Autodesk Fusion 360 part; units mm, degrees
(part 17 of 18)
  line L10453 (179.7854, -37.8851) -> (177.0854, -37.8851)
  line L10454 (177.0854, -39.5851) -> (179.7854, -39.5851)
  line L10455 (177.0854, -37.8851) -> (177.0854, -39.5851)
  line L10456 (103.5852, -77.7106) -> (103.5852, -76.0106)
  line L10457 (100.8852, -76.0106) -> (100.8852, -77.7106)
  line L10458 (100.8852, -77.7106) -> (103.5852, -77.7106)
  line L10459 (103.5852, -76.0106) -> (100.8852, -76.0106)
  line L10460 (103.5852, -56.9478) -> (100.8852, -56.9478)
  line L10461 (103.5852, -58.6478) -> (103.5852, -56.9478)
  line L10462 (100.8852, -56.9478) -> (100.8852, -58.6478)
  line L10463 (100.8852, -58.6478) -> (103.5852, -58.6478)
  line L10464 (103.5852, -20.535) -> (103.5852, -18.835)
  line L10465 (103.5852, -18.835) -> (100.8852, -18.835)
  line L10466 (100.8852, -18.835) -> (100.8852, -20.535)
  line L10467 (100.8852, -20.535) -> (103.5852, -20.535)
  line L10468 (103.5852, -39.5851) -> (103.5852, -37.8851)
  line L10469 (100.8852, -39.5851) -> (103.5852, -39.5851)
  line L10470 (100.8852, -37.8851) -> (100.8852, -39.5851)
  line L10471 (103.5852, -37.8851) -> (100.8852, -37.8851)
  line L10472 (122.6352, -20.535) -> (122.6352, -18.835)
  line L10473 (119.9352, -20.535) -> (122.6352, -20.535)
  line L10474 (122.6352, -18.835) -> (119.9352, -18.835)
  line L10475 (119.9352, -18.835) -> (119.9352, -20.535)
  line L10476 (122.6352, -58.6478) -> (122.6352, -56.9478)
  line L10477 (122.6352, -56.9478) -> (119.9352, -56.9478)
  line L10478 (119.9352, -56.9478) -> (119.9352, -58.6478)
  line L10479 (119.9352, -58.6478) -> (122.6352, -58.6478)
  line L10480 (119.9352, -39.5851) -> (122.6352, -39.5851)
  line L10481 (122.6352, -37.8851) -> (119.9352, -37.8851)
  line L10482 (119.9352, -37.8851) -> (119.9352, -39.5851)
  line L10483 (122.6352, -39.5851) -> (122.6352, -37.8851)
  line L10484 (122.6352, -76.0106) -> (119.9352, -76.0106)
  line L10485 (119.9352, -77.7106) -> (122.6352, -77.7106)
  line L10486 (119.9352, -76.0106) -> (119.9352, -77.7106)
  line L10487 (122.6352, -77.7106) -> (122.6352, -76.0106)
  line L10488 (5.635, -76.0106) -> (5.635, -77.7106)
  line L10489 (8.335, -76.0106) -> (5.635, -76.0106)
  line L10490 (5.635, -77.7106) -> (8.335, -77.7106)
  line L10491 (8.335, -77.7106) -> (8.335, -76.0106)
  line L10492 (24.6851, -77.7106) -> (27.3851, -77.7106)
  line L10493 (24.6851, -76.0106) -> (24.6851, -77.7106)
  line L10494 (27.3851, -76.0106) -> (24.6851, -76.0106)
  line L10495 (27.3851, -77.7106) -> (27.3851, -76.0106)
  line L10496 (43.7351, -77.7106) -> (46.4351, -77.7106)
  line L10497 (46.4351, -77.7106) -> (46.4351, -76.0106)
  line L10498 (43.7351, -76.0106) -> (43.7351, -77.7106)
  line L10499 (46.4351, -76.0106) -> (43.7351, -76.0106)
  line L10500 (62.7851, -18.835) -> (62.7851, -20.535)
  line L10501 (65.4851, -20.535) -> (65.4851, -18.835)
  line L10502 (62.7851, -20.535) -> (65.4851, -20.535)
  line L10503 (65.4851, -18.835) -> (62.7851, -18.835)
  line L10504 (62.7851, -77.7106) -> (65.4851, -77.7106)
  line L10505 (62.7851, -76.0106) -> (62.7851, -77.7106)
  line L10506 (65.4851, -77.7106) -> (65.4851, -76.0106)
  line L10507 (65.4851, -76.0106) -> (62.7851, -76.0106)
  line L10508 (65.4851, -39.5851) -> (65.4851, -37.8851)
  line L10509 (62.7851, -39.5851) -> (65.4851, -39.5851)
  line L10510 (65.4851, -37.8851) -> (62.7851, -37.8851)
  line L10511 (62.7851, -37.8851) -> (62.7851, -39.5851)
  line L10512 (62.7851, -56.9478) -> (62.7851, -58.6478)
  line L10513 (65.4851, -56.9478) -> (62.7851, -56.9478)
  line L10514 (65.4851, -58.6478) -> (65.4851, -56.9478)
  line L10515 (62.7851, -58.6478) -> (65.4851, -58.6478)
  line L10516 (84.5352, -39.5851) -> (84.5352, -37.8851)
  line L10517 (84.5352, -37.8851) -> (81.8352, -37.8851)
  line L10518 (81.8352, -37.8851) -> (81.8352, -39.5851)
  line L10519 (81.8352, -39.5851) -> (84.5352, -39.5851)
  line L10520 (81.8352, -76.0106) -> (81.8352, -77.7106)
  line L10521 (84.5352, -77.7106) -> (84.5352, -76.0106)
  line L10522 (81.8352, -77.7106) -> (84.5352, -77.7106)
  line L10523 (84.5352, -76.0106) -> (81.8352, -76.0106)
  line L10524 (81.8352, -18.835) -> (81.8352, -20.535)
  line L10525 (84.5352, -20.535) -> (84.5352, -18.835)
  line L10526 (84.5352, -18.835) -> (81.8352, -18.835)
  line L10527 (81.8352, -20.535) -> (84.5352, -20.535)
  line L10528 (81.8352, -56.9478) -> (81.8352, -58.6478)
  line L10529 (84.5352, -58.6478) -> (84.5352, -56.9478)
  line L10530 (84.5352, -56.9478) -> (81.8352, -56.9478)
  line L10531 (81.8352, -58.6478) -> (84.5352, -58.6478)
  line L10532 (8.335, -56.9478) -> (5.635, -56.9478)
  line L10533 (5.635, -56.9478) -> (5.635, -58.6478)
  line L10534 (8.335, -58.6478) -> (8.335, -56.9478)
  line L10535 (5.635, -58.6478) -> (8.335, -58.6478)
  line L10536 (8.335, -18.835) -> (5.635, -18.835)
  line L10537 (5.635, -20.535) -> (8.335, -20.535)
  line L10538 (8.335, -20.535) -> (8.335, -18.835)
  line L10539 (5.635, -18.835) -> (5.635, -20.535)
  line L10540 (8.335, -37.8851) -> (5.635, -37.8851)
  line L10541 (8.335, -39.5851) -> (8.335, -37.8851)
  line L10542 (5.635, -37.8851) -> (5.635, -39.5851)
  line L10543 (5.635, -39.5851) -> (8.335, -39.5851)
  line L10544 (27.3851, -37.8851) -> (24.6851, -37.8851)
  line L10545 (24.6851, -37.8851) -> (24.6851, -39.5851)
  line L10546 (27.3851, -39.5851) -> (27.3851, -37.8851)
  line L10547 (24.6851, -39.5851) -> (27.3851, -39.5851)
  line L10548 (27.3851, -18.835) -> (24.6851, -18.835)
  line L10549 (27.3851, -20.535) -> (27.3851, -18.835)
  line L10550 (24.6851, -20.535) -> (27.3851, -20.535)
  line L10551 (24.6851, -18.835) -> (24.6851, -20.535)
  line L10552 (24.6851, -56.9478) -> (24.6851, -58.6478)
  line L10553 (24.6851, -58.6478) -> (27.3851, -58.6478)
  line L10554 (27.3851, -56.9478) -> (24.6851, -56.9478)
  line L10555 (27.3851, -58.6478) -> (27.3851, -56.9478)
  line L10556 (46.4351, -18.835) -> (43.7351, -18.835)
  line L10557 (43.7351, -18.835) -> (43.7351, -20.535)
  line L10558 (46.4351, -20.535) -> (46.4351, -18.835)
  line L10559 (43.7351, -20.535) -> (46.4351, -20.535)
  line L10560 (43.7351, -58.6478) -> (46.4351, -58.6478)
  line L10561 (46.4351, -58.6478) -> (46.4351, -56.9478)
  line L10562 (46.4351, -56.9478) -> (43.7351, -56.9478)
  line L10563 (43.7351, -56.9478) -> (43.7351, -58.6478)
  line L10564 (43.7351, -39.5851) -> (46.4351, -39.5851)
  line L10565 (43.7351, -37.8851) -> (43.7351, -39.5851)
  line L10566 (46.4351, -39.5851) -> (46.4351, -37.8851)
  line L10567 (46.4351, -37.8851) -> (43.7351, -37.8851)
  line L10568 (215.1854, -18.835) -> (215.1854, -20.535)
  line L10569 (217.8854, -18.835) -> (215.1854, -18.835)
  line L10570 (217.8854, -20.535) -> (217.8854, -18.835)
  line L10571 (215.1854, -20.535) -> (217.8854, -20.535)
  line L10572 (217.8854, -76.0106) -> (215.1854, -76.0106)
  line L10573 (217.8854, -77.7106) -> (217.8854, -76.0106)
  line L10574 (215.1854, -77.7106) -> (217.8854, -77.7106)
  line L10575 (215.1854, -76.0106) -> (215.1854, -77.7106)
  line L10576 (215.1854, -58.6478) -> (217.8854, -58.6478)
  line L10577 (217.8854, -56.9478) -> (215.1854, -56.9478)
  line L10578 (217.8854, -58.6478) -> (217.8854, -56.9478)
  line L10579 (215.1854, -56.9478) -> (215.1854, -58.6478)
  line L10580 (215.1854, -37.8851) -> (215.1854, -39.5851)
  line L10581 (217.8854, -39.5851) -> (217.8854, -37.8851)
  line L10582 (215.1854, -39.5851) -> (217.8854, -39.5851)
  line L10583 (217.8854, -37.8851) -> (215.1854, -37.8851)
  line L10584 (196.1354, -37.8851) -> (196.1354, -39.5851)
  line L10585 (196.1354, -39.5851) -> (198.8354, -39.5851)
  line L10586 (198.8354, -39.5851) -> (198.8354, -37.8851)
  line L10587 (198.8354, -37.8851) -> (196.1354, -37.8851)
  line L10588 (198.8354, -76.0106) -> (196.1354, -76.0106)
  line L10589 (198.8354, -77.7106) -> (198.8354, -76.0106)
  line L10590 (196.1354, -76.0106) -> (196.1354, -77.7106)
  line L10591 (196.1354, -77.7106) -> (198.8354, -77.7106)
  line L10592 (196.1354, -56.9478) -> (196.1354, -58.6478)
  line L10593 (196.1354, -58.6478) -> (198.8354, -58.6478)
  line L10594 (198.8354, -56.9478) -> (196.1354, -56.9478)
  line L10595 (198.8354, -58.6478) -> (198.8354, -56.9478)
  line L10596 (196.1354, -18.835) -> (196.1354, -20.535)
  line L10597 (196.1354, -20.535) -> (198.8354, -20.535)
  line L10598 (198.8354, -18.835) -> (196.1354, -18.835)
  line L10599 (198.8354, -20.535) -> (198.8354, -18.835)
  line L10600 (203.2384, -4.21) -> (201.6384, -4.21)
  line L10601 (201.6384, -4.21) -> (201.6384, -3.41)
  line L10602 (201.6384, -3.41) -> (203.2384, -3.41)
  line L10603 (203.2384, -3.41) -> (203.2384, -4.21)
  line L10604 (199.7334, -7.131) -> (199.7334, -6.331)
  line L10605 (199.7334, -6.331) -> (201.3334, -6.331)
  line L10606 (201.3334, -7.131) -> (199.7334, -7.131)
  line L10607 (201.3334, -6.331) -> (201.3334, -7.131)
  line L10608 (206.5404, -4.426) -> (206.5404, -5.226)
  line L10609 (204.9404, -4.426) -> (206.5404, -4.426)
  line L10610 (206.5404, -5.226) -> (204.9404, -5.226)
  line L10611 (204.9404, -5.226) -> (204.9404, -4.426)
  line L10612 (-5.7371, 1.189) -> (10.5631, 1.189)
  line L10613 (10.5631, -12.111) -> (-5.7371, -12.111)
  line L10614 (-5.7371, -12.111) -> (-5.7371, 1.189)
  line L10615 (10.5631, 1.189) -> (10.5631, -12.111)
  line L10616 (196.9574, -3.429) -> (196.9574, -5.529)
  line L10617 (195.7074, -5.529) -> (195.7074, -3.429)
  line L10618 (195.7074, -3.429) -> (196.9574, -3.429)
  line L10619 (196.9574, -5.529) -> (195.7074, -5.529)
  line L10620 (177.1673, -5.588) -> (172.3373, -5.588)
  line L10621 (172.3373, -3.048) -> (177.1673, -3.048)
  line L10622 (172.3373, -5.588) -> (172.3373, -3.048)
  line L10623 (177.1673, -3.048) -> (177.1673, -5.588)
  line L10624 (199.8604, -1.505) -> (201.4604, -1.505)
  line L10625 (201.4604, -1.505) -> (201.4604, -2.305)
  line L10626 (201.4604, -2.305) -> (199.8604, -2.305)
  line L10627 (199.8604, -2.305) -> (199.8604, -1.505)
  line L10628 (214.5745, -5.2629) -> (214.5745, -12.2629)
  line L10629 (214.5745, -12.2629) -> (207.5745, -12.2629)
  line L10630 (207.5745, -5.2629) -> (214.5745, -5.2629)
  line L10631 (207.5745, -12.2629) -> (207.5745, -5.2629)
  line L10632 (188.5064, -6.331) -> (188.5064, -7.131)
  line L10633 (186.9064, -6.331) -> (188.5064, -6.331)
  line L10634 (188.5064, -7.131) -> (186.9064, -7.131)
  line L10635 (186.9064, -7.131) -> (186.9064, -6.331)
  line L10636 (182.3344, -7.131) -> (182.3344, -6.331)
  line L10637 (183.9344, -7.131) -> (182.3344, -7.131)
  line L10638 (183.9344, -6.331) -> (183.9344, -7.131)
  line L10639 (182.3344, -6.331) -> (183.9344, -6.331)
  line L10640 (208.6854, -0.786) -> (211.6854, -0.786)
  line L10641 (208.6854, -3.786) -> (208.6854, -0.786)
  line L10642 (211.6854, -3.786) -> (208.6854, -3.786)
  line L10643 (211.6854, -0.786) -> (211.6854, -3.786)
  line L10644 (138.9853, -77.7106) -> (141.6853, -77.7106)
  line L10645 (138.9853, -76.0106) -> (138.9853, -77.7106)
  line L10646 (141.6853, -76.0106) -> (138.9853, -76.0106)
  line L10647 (141.6853, -77.7106) -> (141.6853, -76.0106)
  line L10648 (138.9853, -20.535) -> (141.6853, -20.535)
  line L10649 (141.6853, -20.535) -> (141.6853, -18.835)
  line L10650 (141.6853, -18.835) -> (138.9853, -18.835)
  line L10651 (138.9853, -18.835) -> (138.9853, -20.535)
  line L10652 (138.9853, -39.5851) -> (141.6853, -39.5851)
  line L10653 (141.6853, -37.8851) -> (138.9853, -37.8851)
  line L10654 (138.9853, -37.8851) -> (138.9853, -39.5851)
  line L10655 (141.6853, -39.5851) -> (141.6853, -37.8851)
  line L10656 (138.9853, -56.9478) -> (138.9853, -58.6478)
  line L10657 (141.6853, -56.9478) -> (138.9853, -56.9478)
  line L10658 (138.9853, -58.6478) -> (141.6853, -58.6478)
  line L10659 (141.6853, -58.6478) -> (141.6853, -56.9478)
  line L10660 (158.0353, -20.535) -> (160.7353, -20.535)
  line L10661 (160.7353, -18.835) -> (158.0353, -18.835)
  line L10662 (160.7353, -20.535) -> (160.7353, -18.835)
  line L10663 (158.0353, -18.835) -> (158.0353, -20.535)
  line L10664 (158.0353, -76.0106) -> (158.0353, -77.7106)
  line L10665 (160.7353, -76.0106) -> (158.0353, -76.0106)
  line L10666 (158.0353, -77.7106) -> (160.7353, -77.7106)
  line L10667 (160.7353, -77.7106) -> (160.7353, -76.0106)
  line L10668 (158.0353, -56.9478) -> (158.0353, -58.6478)
  line L10669 (160.7353, -58.6478) -> (160.7353, -56.9478)
  line L10670 (160.7353, -56.9478) -> (158.0353, -56.9478)
  line L10671 (158.0353, -58.6478) -> (160.7353, -58.6478)
  line L10672 (160.7353, -39.5851) -> (160.7353, -37.8851)
  line L10673 (160.7353, -37.8851) -> (158.0353, -37.8851)
  line L10674 (158.0353, -39.5851) -> (160.7353, -39.5851)
  line L10675 (158.0353, -37.8851) -> (158.0353, -39.5851)
  line L10676 (177.0854, -20.535) -> (179.7854, -20.535)
  line L10677 (179.7854, -18.835) -> (177.0854, -18.835)
  line L10678 (179.7854, -20.535) -> (179.7854, -18.835)
  line L10679 (177.0854, -18.835) -> (177.0854, -20.535)
  line L10680 (177.0854, -76.0106) -> (177.0854, -77.7106)
  line L10681 (179.7854, -77.7106) -> (179.7854, -76.0106)
  line L10682 (177.0854, -77.7106) -> (179.7854, -77.7106)
  line L10683 (179.7854, -76.0106) -> (177.0854, -76.0106)
  line L10684 (177.0854, -56.9478) -> (177.0854, -58.6478)
  line L10685 (177.0854, -58.6478) -> (179.7854, -58.6478)
  line L10686 (179.7854, -58.6478) -> (179.7854, -56.9478)
  line L10687 (179.7854, -56.9478) -> (177.0854, -56.9478)
  line L10688 (177.0854, -37.8851) -> (177.0854, -39.5851)
  line L10689 (177.0854, -39.5851) -> (179.7854, -39.5851)
  line L10690 (179.7854, -39.5851) -> (179.7854, -37.8851)
  line L10691 (179.7854, -37.8851) -> (177.0854, -37.8851)
  line L10692 (103.5852, -77.7106) -> (103.5852, -76.0106)
  line L10693 (100.8852, -76.0106) -> (100.8852, -77.7106)
  line L10694 (103.5852, -76.0106) -> (100.8852, -76.0106)
  line L10695 (100.8852, -77.7106) -> (103.5852, -77.7106)
  line L10696 (103.5852, -58.6478) -> (103.5852, -56.9478)
  line L10697 (103.5852, -56.9478) -> (100.8852, -56.9478)
  line L10698 (100.8852, -56.9478) -> (100.8852, -58.6478)
  line L10699 (100.8852, -58.6478) -> (103.5852, -58.6478)
  line L10700 (100.8852, -20.535) -> (103.5852, -20.535)
  line L10701 (100.8852, -18.835) -> (100.8852, -20.535)
  line L10702 (103.5852, -20.535) -> (103.5852, -18.835)
  line L10703 (103.5852, -18.835) -> (100.8852, -18.835)
  line L10704 (103.5852, -39.5851) -> (103.5852, -37.8851)
  line L10705 (100.8852, -37.8851) -> (100.8852, -39.5851)
  line L10706 (100.8852, -39.5851) -> (103.5852, -39.5851)
  line L10707 (103.5852, -37.8851) -> (100.8852, -37.8851)
  line L10708 (122.6352, -18.835) -> (119.9352, -18.835)
  line L10709 (119.9352, -18.835) -> (119.9352, -20.535)
  line L10710 (119.9352, -20.535) -> (122.6352, -20.535)
  line L10711 (122.6352, -20.535) -> (122.6352, -18.835)
  line L10712 (119.9352, -58.6478) -> (122.6352, -58.6478)
  line L10713 (122.6352, -56.9478) -> (119.9352, -56.9478)
  line L10714 (122.6352, -58.6478) -> (122.6352, -56.9478)
  line L10715 (119.9352, -56.9478) -> (119.9352, -58.6478)
  line L10716 (122.6352, -39.5851) -> (122.6352, -37.8851)
  line L10717 (119.9352, -39.5851) -> (122.6352, -39.5851)
  line L10718 (119.9352, -37.8851) -> (119.9352, -39.5851)
  line L10719 (122.6352, -37.8851) -> (119.9352, -37.8851)
  line L10720 (122.6352, -76.0106) -> (119.9352, -76.0106)
  line L10721 (122.6352, -77.7106) -> (122.6352, -76.0106)
  line L10722 (119.9352, -76.0106) -> (119.9352, -77.7106)
  line L10723 (119.9352, -77.7106) -> (122.6352, -77.7106)
  line L10724 (5.635, -76.0106) -> (5.635, -77.7106)
  line L10725 (8.335, -77.7106) -> (8.335, -76.0106)
  line L10726 (5.635, -77.7106) -> (8.335, -77.7106)
  line L10727 (8.335, -76.0106) -> (5.635, -76.0106)
  line L10728 (27.3851, -76.0106) -> (24.6851, -76.0106)
  line L10729 (27.3851, -77.7106) -> (27.3851, -76.0106)
  line L10730 (24.6851, -76.0106) -> (24.6851, -77.7106)
  line L10731 (24.6851, -77.7106) -> (27.3851, -77.7106)
  line L10732 (46.4351, -76.0106) -> (43.7351, -76.0106)
  line L10733 (43.7351, -77.7106) -> (46.4351, -77.7106)
  line L10734 (46.4351, -77.7106) -> (46.4351, -76.0106)
  line L10735 (43.7351, -76.0106) -> (43.7351, -77.7106)
  line L10736 (62.7851, -20.535) -> (65.4851, -20.535)
  line L10737 (65.4851, -20.535) -> (65.4851, -18.835)
  line L10738 (62.7851, -18.835) -> (62.7851, -20.535)
  line L10739 (65.4851, -18.835) -> (62.7851, -18.835)
  line L10740 (62.7851, -76.0106) -> (62.7851, -77.7106)
  line L10741 (65.4851, -76.0106) -> (62.7851, -76.0106)
  line L10742 (62.7851, -77.7106) -> (65.4851, -77.7106)
  line L10743 (65.4851, -77.7106) -> (65.4851, -76.0106)
  line L10744 (62.7851, -39.5851) -> (65.4851, -39.5851)
  line L10745 (65.4851, -39.5851) -> (65.4851, -37.8851)
  line L10746 (65.4851, -37.8851) -> (62.7851, -37.8851)
  line L10747 (62.7851, -37.8851) -> (62.7851, -39.5851)
  line L10748 (62.7851, -58.6478) -> (65.4851, -58.6478)
  line L10749 (62.7851, -56.9478) -> (62.7851, -58.6478)
  line L10750 (65.4851, -58.6478) -> (65.4851, -56.9478)
  line L10751 (65.4851, -56.9478) -> (62.7851, -56.9478)
  line L10752 (84.5352, -39.5851) -> (84.5352, -37.8851)
  line L10753 (81.8352, -37.8851) -> (81.8352, -39.5851)
  line L10754 (81.8352, -39.5851) -> (84.5352, -39.5851)
  line L10755 (84.5352, -37.8851) -> (81.8352, -37.8851)
  line L10756 (84.5352, -77.7106) -> (84.5352, -76.0106)
  line L10757 (81.8352, -76.0106) -> (81.8352, -77.7106)
  line L10758 (81.8352, -77.7106) -> (84.5352, -77.7106)
  line L10759 (84.5352, -76.0106) -> (81.8352, -76.0106)
  line L10760 (84.5352, -20.535) -> (84.5352, -18.835)
  line L10761 (84.5352, -18.835) -> (81.8352, -18.835)
  line L10762 (81.8352, -20.535) -> (84.5352, -20.535)
  line L10763 (81.8352, -18.835) -> (81.8352, -20.535)
  line L10764 (81.8352, -58.6478) -> (84.5352, -58.6478)
  line L10765 (81.8352, -56.9478) -> (81.8352, -58.6478)
  line L10766 (84.5352, -56.9478) -> (81.8352, -56.9478)
  line L10767 (84.5352, -58.6478) -> (84.5352, -56.9478)
  line L10768 (5.635, -58.6478) -> (8.335, -58.6478)
  line L10769 (8.335, -56.9478) -> (5.635, -56.9478)
  line L10770 (5.635, -56.9478) -> (5.635, -58.6478)
  line L10771 (8.335, -58.6478) -> (8.335, -56.9478)
  line L10772 (8.335, -20.535) -> (8.335, -18.835)
  line L10773 (8.335, -18.835) -> (5.635, -18.835)
  line L10774 (5.635, -18.835) -> (5.635, -20.535)
  line L10775 (5.635, -20.535) -> (8.335, -20.535)
  line L10776 (8.335, -37.8851) -> (5.635, -37.8851)
  line L10777 (5.635, -39.5851) -> (8.335, -39.5851)
  line L10778 (5.635, -37.8851) -> (5.635, -39.5851)
  line L10779 (8.335, -39.5851) -> (8.335, -37.8851)
  line L10780 (27.3851, -37.8851) -> (24.6851, -37.8851)
  line L10781 (24.6851, -39.5851) -> (27.3851, -39.5851)
  line L10782 (24.6851, -37.8851) -> (24.6851, -39.5851)
  line L10783 (27.3851, -39.5851) -> (27.3851, -37.8851)
  line L10784 (24.6851, -20.535) -> (27.3851, -20.535)
  line L10785 (27.3851, -20.535) -> (27.3851, -18.835)
  line L10786 (24.6851, -18.835) -> (24.6851, -20.535)
  line L10787 (27.3851, -18.835) -> (24.6851, -18.835)
  line L10788 (24.6851, -56.9478) -> (24.6851, -58.6478)
  line L10789 (27.3851, -56.9478) -> (24.6851, -56.9478)
  line L10790 (24.6851, -58.6478) -> (27.3851, -58.6478)
  line L10791 (27.3851, -58.6478) -> (27.3851, -56.9478)
  line L10792 (43.7351, -20.535) -> (46.4351, -20.535)
  line L10793 (43.7351, -18.835) -> (43.7351, -20.535)
  line L10794 (46.4351, -20.535) -> (46.4351, -18.835)
  line L10795 (46.4351, -18.835) -> (43.7351, -18.835)
  line L10796 (43.7351, -58.6478) -> (46.4351, -58.6478)
  line L10797 (46.4351, -58.6478) -> (46.4351, -56.9478)
  line L10798 (46.4351, -56.9478) -> (43.7351, -56.9478)
  line L10799 (43.7351, -56.9478) -> (43.7351, -58.6478)
  line L10800 (46.4351, -37.8851) -> (43.7351, -37.8851)
  line L10801 (43.7351, -39.5851) -> (46.4351, -39.5851)
  line L10802 (43.7351, -37.8851) -> (43.7351, -39.5851)
  line L10803 (46.4351, -39.5851) -> (46.4351, -37.8851)
  line L10804 (217.8854, -20.535) -> (217.8854, -18.835)
  line L10805 (217.8854, -18.835) -> (215.1854, -18.835)
  line L10806 (215.1854, -18.835) -> (215.1854, -20.535)
  line L10807 (215.1854, -20.535) -> (217.8854, -20.535)
  line L10808 (215.1854, -77.7106) -> (217.8854, -77.7106)
  line L10809 (215.1854, -76.0106) -> (215.1854, -77.7106)
  line L10810 (217.8854, -76.0106) -> (215.1854, -76.0106)
  line L10811 (217.8854, -77.7106) -> (217.8854, -76.0106)
  line L10812 (217.8854, -56.9478) -> (215.1854, -56.9478)
  line L10813 (215.1854, -58.6478) -> (217.8854, -58.6478)
  line L10814 (217.8854, -58.6478) -> (217.8854, -56.9478)
  line L10815 (215.1854, -56.9478) -> (215.1854, -58.6478)
  line L10816 (217.8854, -37.8851) -> (215.1854, -37.8851)
  line L10817 (215.1854, -37.8851) -> (215.1854, -39.5851)
  line L10818 (217.8854, -39.5851) -> (217.8854, -37.8851)
  line L10819 (215.1854, -39.5851) -> (217.8854, -39.5851)
  line L10820 (198.8354, -37.8851) -> (196.1354, -37.8851)
  line L10821 (196.1354, -37.8851) -> (196.1354, -39.5851)
  line L10822 (196.1354, -39.5851) -> (198.8354, -39.5851)
  line L10823 (198.8354, -39.5851) -> (198.8354, -37.8851)
  line L10824 (196.1354, -77.7106) -> (198.8354, -77.7106)
  line L10825 (196.1354, -76.0106) -> (196.1354, -77.7106)
  line L10826 (198.8354, -76.0106) -> (196.1354, -76.0106)
  line L10827 (198.8354, -77.7106) -> (198.8354, -76.0106)
  line L10828 (196.1354, -58.6478) -> (198.8354, -58.6478)
  line L10829 (196.1354, -56.9478) -> (196.1354, -58.6478)
  line L10830 (198.8354, -58.6478) -> (198.8354, -56.9478)
  line L10831 (198.8354, -56.9478) -> (196.1354, -56.9478)
  line L10832 (198.8354, -20.535) -> (198.8354, -18.835)
  line L10833 (196.1354, -20.535) -> (198.8354, -20.535)
  line L10834 (198.8354, -18.835) -> (196.1354, -18.835)
  line L10835 (196.1354, -18.835) -> (196.1354, -20.535)
  line L10836 (201.6384, -3.41) -> (203.2384, -3.41)
  line L10837 (201.6384, -4.21) -> (201.6384, -3.41)
  line L10838 (203.2384, -3.41) -> (203.2384, -4.21)
  line L10839 (203.2384, -4.21) -> (201.6384, -4.21)
  line L10840 (199.7334, -6.331) -> (201.3334, -6.331)
  line L10841 (201.3334, -7.131) -> (199.7334, -7.131)
  line L10842 (199.7334, -7.131) -> (199.7334, -6.331)
  line L10843 (201.3334, -6.331) -> (201.3334, -7.131)
  line L10844 (204.9404, -4.426) -> (206.5404, -4.426)
  line L10845 (206.5404, -4.426) -> (206.5404, -5.226)
  line L10846 (204.9404, -5.226) -> (204.9404, -4.426)
  line L10847 (206.5404, -5.226) -> (204.9404, -5.226)
  line L10848 (-5.7371, -12.111) -> (-5.7371, 1.189)
  line L10849 (10.5631, 1.189) -> (10.5631, -12.111)
  line L10850 (10.5631, -12.111) -> (-5.7371, -12.111)
  line L10851 (-5.7371, 1.189) -> (10.5631, 1.189)
  line L10852 (195.7074, -5.529) -> (195.7074, -3.429)
  line L10853 (195.7074, -3.429) -> (196.9574, -3.429)
  line L10854 (196.9574, -5.529) -> (195.7074, -5.529)
  line L10855 (196.9574, -3.429) -> (196.9574, -5.529)
  line L10856 (177.1673, -5.588) -> (172.3373, -5.588)
  line L10857 (177.1673, -3.048) -> (177.1673, -5.588)
  line L10858 (172.3373, -3.048) -> (177.1673, -3.048)
  line L10859 (172.3373, -5.588) -> (172.3373, -3.048)
  line L10860 (208.2754, -3.1661) -> (208.6954, -3.1661)
  line L10861 (208.6954, -3.1661) -> (208.6954, -3.4061)
  line L10862 (208.6954, -3.4061) -> (208.2754, -3.4061)
  line L10863 (208.2754, -3.4061) -> (208.2754, -3.1661)
  line L10864 (208.6954, -2.666) -> (208.6954, -2.906)
  line L10865 (208.2754, -2.666) -> (208.6954, -2.666)
  line L10866 (208.2754, -2.906) -> (208.2754, -2.666)
  line L10867 (208.6954, -2.906) -> (208.2754, -2.906)
  line L10868 (208.2754, -2.1659) -> (208.6954, -2.1659)
  line L10869 (208.2754, -2.4059) -> (208.2754, -2.1659)
  line L10870 (208.6954, -2.1659) -> (208.6954, -2.4059)
  line L10871 (208.6954, -2.4059) -> (208.2754, -2.4059)
  line L10872 (208.2754, -1.906) -> (208.2754, -1.666)
  line L10873 (208.2754, -1.666) -> (208.6954, -1.666)
  line L10874 (208.6954, -1.666) -> (208.6954, -1.906)
  line L10875 (208.6954, -1.906) -> (208.2754, -1.906)
  line L10876 (208.6954, -1.4061) -> (208.2754, -1.4061)
  line L10877 (208.2754, -1.4061) -> (208.2754, -1.1661)
  line L10878 (208.6954, -1.1661) -> (208.6954, -1.4061)
  line L10879 (208.2754, -1.1661) -> (208.6954, -1.1661)
  line L10880 (212.0954, -1.4059) -> (211.6754, -1.4059)
  line L10881 (211.6754, -1.1659) -> (212.0954, -1.1659)
  line L10882 (212.0954, -1.1659) -> (212.0954, -1.4059)
  line L10883 (211.6754, -1.4059) -> (211.6754, -1.1659)
  line L10884 (211.6754, -1.906) -> (211.6754, -1.666)
  line L10885 (212.0954, -1.906) -> (211.6754, -1.906)
  line L10886 (212.0954, -1.666) -> (212.0954, -1.906)
  line L10887 (211.6754, -1.666) -> (212.0954, -1.666)
  line L10888 (212.0954, -2.4061) -> (211.6754, -2.4061)
  line L10889 (212.0954, -2.1661) -> (212.0954, -2.4061)
  line L10890 (211.6754, -2.4061) -> (211.6754, -2.1661)
  line L10891 (211.6754, -2.1661) -> (212.0954, -2.1661)
  line L10892 (211.6754, -2.666) -> (212.0954, -2.666)
  line L10893 (212.0954, -2.666) -> (212.0954, -2.906)
  line L10894 (211.6754, -2.906) -> (211.6754, -2.666)
  line L10895 (212.0954, -2.906) -> (211.6754, -2.906)
  line L10896 (211.6754, -3.4059) -> (211.6754, -3.1659)
  line L10897 (211.6754, -3.1659) -> (212.0954, -3.1659)
  line L10898 (212.0954, -3.1659) -> (212.0954, -3.4059)
  line L10899 (212.0954, -3.4059) -> (211.6754, -3.4059)
  line L10900 (138.7753, -77.1606) -> (138.9953, -77.1606)
  line L10901 (138.7753, -76.5606) -> (138.7753, -77.1606)
  line L10902 (138.9953, -76.5606) -> (138.7753, -76.5606)
  line L10903 (138.9953, -77.1606) -> (138.9953, -76.5606)
  line L10904 (141.6753, -76.5606) -> (141.8953, -76.5606)
  line L10905 (141.6753, -77.1606) -> (141.6753, -76.5606)
  line L10906 (141.8953, -77.1606) -> (141.6753, -77.1606)
  line L10907 (141.8953, -76.5606) -> (141.8953, -77.1606)
  line L10908 (138.7753, -19.385) -> (138.7753, -19.985)
  line L10909 (138.9953, -19.385) -> (138.7753, -19.385)
  line L10910 (138.9953, -19.985) -> (138.9953, -19.385)
  line L10911 (138.7753, -19.985) -> (138.9953, -19.985)
  line L10912 (141.8953, -19.985) -> (141.6753, -19.985)
  line L10913 (141.6753, -19.385) -> (141.8953, -19.385)
  line L10914 (141.6753, -19.985) -> (141.6753, -19.385)
  line L10915 (141.8953, -19.385) -> (141.8953, -19.985)
  line L10916 (138.7753, -39.0351) -> (138.9953, -39.0351)
  line L10917 (138.9953, -39.0351) -> (138.9953, -38.4351)
  line L10918 (138.7753, -38.4351) -> (138.7753, -39.0351)
  line L10919 (138.9953, -38.4351) -> (138.7753, -38.4351)
  line L10920 (141.6753, -38.4351) -> (141.8953, -38.4351)
  line L10921 (141.6753, -39.0351) -> (141.6753, -38.4351)
  line L10922 (141.8953, -38.4351) -> (141.8953, -39.0351)
  line L10923 (141.8953, -39.0351) -> (141.6753, -39.0351)
  line L10924 (138.9953, -57.4978) -> (138.7753, -57.4978)
  line L10925 (138.9953, -58.0978) -> (138.9953, -57.4978)
  line L10926 (138.7753, -58.0978) -> (138.9953, -58.0978)
  line L10927 (138.7753, -57.4978) -> (138.7753, -58.0978)
  line L10928 (141.8953, -58.0978) -> (141.6753, -58.0978)
  line L10929 (141.8953, -57.4978) -> (141.8953, -58.0978)
  line L10930 (141.6753, -57.4978) -> (141.8953, -57.4978)
  line L10931 (141.6753, -58.0978) -> (141.6753, -57.4978)
  line L10932 (158.0453, -19.385) -> (157.8253, -19.385)
  line L10933 (157.8253, -19.385) -> (157.8253, -19.985)
  line L10934 (157.8253, -19.985) -> (158.0453, -19.985)
  line L10935 (158.0453, -19.985) -> (158.0453, -19.385)
  line L10936 (160.9453, -19.985) -> (160.7253, -19.985)
  line L10937 (160.7253, -19.985) -> (160.7253, -19.385)
  line L10938 (160.7253, -19.385) -> (160.9453, -19.385)
  line L10939 (160.9453, -19.385) -> (160.9453, -19.985)
  line L10940 (158.0453, -76.5606) -> (157.8253, -76.5606)
  line L10941 (158.0453, -77.1606) -> (158.0453, -76.5606)
  line L10942 (157.8253, -76.5606) -> (157.8253, -77.1606)
  line L10943 (157.8253, -77.1606) -> (158.0453, -77.1606)
  line L10944 (160.7253, -77.1606) -> (160.7253, -76.5606)
  line L10945 (160.9453, -77.1606) -> (160.7253, -77.1606)
  line L10946 (160.7253, -76.5606) -> (160.9453, -76.5606)
  line L10947 (160.9453, -76.5606) -> (160.9453, -77.1606)
  line L10948 (158.0453, -58.0978) -> (158.0453, -57.4978)
  line L10949 (158.0453, -57.4978) -> (157.8253, -57.4978)
  line L10950 (157.8253, -58.0978) -> (158.0453, -58.0978)
  line L10951 (157.8253, -57.4978) -> (157.8253, -58.0978)
  line L10952 (160.7253, -58.0978) -> (160.7253, -57.4978)
  line L10953 (160.7253, -57.4978) -> (160.9453, -57.4978)
  line L10954 (160.9453, -58.0978) -> (160.7253, -58.0978)
  line L10955 (160.9453, -57.4978) -> (160.9453, -58.0978)
  line L10956 (158.0453, -39.0351) -> (158.0453, -38.4351)
  line L10957 (157.8253, -39.0351) -> (158.0453, -39.0351)
  line L10958 (158.0453, -38.4351) -> (157.8253, -38.4351)
  line L10959 (157.8253, -38.4351) -> (157.8253, -39.0351)
  line L10960 (160.7253, -38.4351) -> (160.9453, -38.4351)
  line L10961 (160.9453, -38.4351) -> (160.9453, -39.0351)
  line L10962 (160.9453, -39.0351) -> (160.7253, -39.0351)
  line L10963 (160.7253, -39.0351) -> (160.7253, -38.4351)
  line L10964 (177.0954, -19.985) -> (177.0954, -19.385)
  line L10965 (176.8754, -19.985) -> (177.0954, -19.985)
  line L10966 (176.8754, -19.385) -> (176.8754, -19.985)
  line L10967 (177.0954, -19.385) -> (176.8754, -19.385)
  line L10968 (179.9954, -19.985) -> (179.7754, -19.985)
  line L10969 (179.7754, -19.985) -> (179.7754, -19.385)
  line L10970 (179.7754, -19.385) -> (179.9954, -19.385)
  line L10971 (179.9954, -19.385) -> (179.9954, -19.985)
  line L10972 (176.8754, -76.5606) -> (176.8754, -77.1606)
  line L10973 (177.0954, -76.5606) -> (176.8754, -76.5606)
  line L10974 (176.8754, -77.1606) -> (177.0954, -77.1606)
  line L10975 (177.0954, -77.1606) -> (177.0954, -76.5606)
  line L10976 (179.9954, -77.1606) -> (179.7754, -77.1606)
  line L10977 (179.7754, -76.5606) -> (179.9954, -76.5606)
  line L10978 (179.7754, -77.1606) -> (179.7754, -76.5606)
  line L10979 (179.9954, -76.5606) -> (179.9954, -77.1606)
  line L10980 (177.0954, -57.4978) -> (176.8754, -57.4978)
  line L10981 (176.8754, -58.0978) -> (177.0954, -58.0978)
  line L10982 (176.8754, -57.4978) -> (176.8754, -58.0978)
  line L10983 (177.0954, -58.0978) -> (177.0954, -57.4978)
  line L10984 (179.7754, -57.4978) -> (179.9954, -57.4978)
  line L10985 (179.7754, -58.0978) -> (179.7754, -57.4978)
  line L10986 (179.9954, -57.4978) -> (179.9954, -58.0978)
  line L10987 (179.9954, -58.0978) -> (179.7754, -58.0978)
  line L10988 (177.0954, -39.0351) -> (177.0954, -38.4351)
  line L10989 (176.8754, -39.0351) -> (177.0954, -39.0351)
  line L10990 (176.8754, -38.4351) -> (176.8754, -39.0351)
  line L10991 (177.0954, -38.4351) -> (176.8754, -38.4351)
  line L10992 (179.9954, -38.4351) -> (179.9954, -39.0351)
  line L10993 (179.7754, -38.4351) -> (179.9954, -38.4351)
  line L10994 (179.7754, -39.0351) -> (179.7754, -38.4351)
  line L10995 (179.9954, -39.0351) -> (179.7754, -39.0351)
  line L10996 (100.6752, -76.5606) -> (100.6752, -77.1606)
  line L10997 (100.8952, -77.1606) -> (100.8952, -76.5606)
  line L10998 (100.6752, -77.1606) -> (100.8952, -77.1606)
  line L10999 (100.8952, -76.5606) -> (100.6752, -76.5606)
  line L11000 (103.7952, -77.1606) -> (103.5752, -77.1606)
  line L11001 (103.5752, -77.1606) -> (103.5752, -76.5606)
  line L11002 (103.7952, -76.5606) -> (103.7952, -77.1606)
  line L11003 (103.5752, -76.5606) -> (103.7952, -76.5606)
  line L11004 (100.8952, -57.4978) -> (100.6752, -57.4978)
  line L11005 (100.8952, -58.0978) -> (100.8952, -57.4978)
  line L11006 (100.6752, -58.0978) -> (100.8952, -58.0978)
  line L11007 (100.6752, -57.4978) -> (100.6752, -58.0978)
  line L11008 (103.7952, -57.4978) -> (103.7952, -58.0978)
  line L11009 (103.5752, -58.0978) -> (103.5752, -57.4978)
  line L11010 (103.7952, -58.0978) -> (103.5752, -58.0978)
  line L11011 (103.5752, -57.4978) -> (103.7952, -57.4978)
  line L11012 (100.6752, -19.385) -> (100.6752, -19.985)
  line L11013 (100.8952, -19.985) -> (100.8952, -19.385)
  line L11014 (100.6752, -19.985) -> (100.8952, -19.985)
  line L11015 (100.8952, -19.385) -> (100.6752, -19.385)
  line L11016 (103.5752, -19.385) -> (103.7952, -19.385)
  line L11017 (103.5752, -19.985) -> (103.5752, -19.385)
  line L11018 (103.7952, -19.985) -> (103.5752, -19.985)
  line L11019 (103.7952, -19.385) -> (103.7952, -19.985)
  line L11020 (100.8952, -38.4351) -> (100.6752, -38.4351)
  line L11021 (100.6752, -38.4351) -> (100.6752, -39.0351)
  line L11022 (100.8952, -39.0351) -> (100.8952, -38.4351)
  line L11023 (100.6752, -39.0351) -> (100.8952, -39.0351)
  line L11024 (103.7952, -39.0351) -> (103.5752, -39.0351)
  line L11025 (103.5752, -38.4351) -> (103.7952, -38.4351)
  line L11026 (103.5752, -39.0351) -> (103.5752, -38.4351)
  line L11027 (103.7952, -38.4351) -> (103.7952, -39.0351)
  line L11028 (119.9452, -19.385) -> (119.7252, -19.385)
  line L11029 (119.9452, -19.985) -> (119.9452, -19.385)
  line L11030 (119.7252, -19.385) -> (119.7252, -19.985)
  line L11031 (119.7252, -19.985) -> (119.9452, -19.985)
  line L11032 (122.6252, -19.985) -> (122.6252, -19.385)
  line L11033 (122.8452, -19.385) -> (122.8452, -19.985)
  line L11034 (122.6252, -19.385) -> (122.8452, -19.385)
  line L11035 (122.8452, -19.985) -> (122.6252, -19.985)
  line L11036 (119.9452, -58.0978) -> (119.9452, -57.4978)
  line L11037 (119.9452, -57.4978) -> (119.7252, -57.4978)
  line L11038 (119.7252, -57.4978) -> (119.7252, -58.0978)
  line L11039 (119.7252, -58.0978) -> (119.9452, -58.0978)
  line L11040 (122.8452, -58.0978) -> (122.6252, -58.0978)
  line L11041 (122.6252, -58.0978) -> (122.6252, -57.4978)
  line L11042 (122.6252, -57.4978) -> (122.8452, -57.4978)
  line L11043 (122.8452, -57.4978) -> (122.8452, -58.0978)
  line L11044 (119.9452, -39.0351) -> (119.9452, -38.4351)
  line L11045 (119.9452, -38.4351) -> (119.7252, -38.4351)
  line L11046 (119.7252, -38.4351) -> (119.7252, -39.0351)
  line L11047 (119.7252, -39.0351) -> (119.9452, -39.0351)
  line L11048 (122.8452, -39.0351) -> (122.6252, -39.0351)
  line L11049 (122.6252, -38.4351) -> (122.8452, -38.4351)
  line L11050 (122.6252, -39.0351) -> (122.6252, -38.4351)
  line L11051 (122.8452, -38.4351) -> (122.8452, -39.0351)
  line L11052 (119.7252, -76.5606) -> (119.7252, -77.1606)
  line L11053 (119.9452, -76.5606) -> (119.7252, -76.5606)
  line L11054 (119.9452, -77.1606) -> (119.9452, -76.5606)
  line L11055 (119.7252, -77.1606) -> (119.9452, -77.1606)
  line L11056 (122.8452, -77.1606) -> (122.6252, -77.1606)
  line L11057 (122.6252, -77.1606) -> (122.6252, -76.5606)
  line L11058 (122.8452, -76.5606) -> (122.8452, -77.1606)
  line L11059 (122.6252, -76.5606) -> (122.8452, -76.5606)
  line L11060 (5.645, -76.5606) -> (5.425, -76.5606)
  line L11061 (5.425, -76.5606) -> (5.425, -77.1606)
  line L11062 (5.425, -77.1606) -> (5.645, -77.1606)
  line L11063 (5.645, -77.1606) -> (5.645, -76.5606)
  line L11064 (8.325, -77.1606) -> (8.325, -76.5606)
  line L11065 (8.545, -76.5606) -> (8.545, -77.1606)
  line L11066 (8.545, -77.1606) -> (8.325, -77.1606)
  line L11067 (8.325, -76.5606) -> (8.545, -76.5606)
  line L11068 (24.6951, -76.5606) -> (24.4751, -76.5606)
  line L11069 (24.6951, -77.1606) -> (24.6951, -76.5606)
  line L11070 (24.4751, -76.5606) -> (24.4751, -77.1606)
  line L11071 (24.4751, -77.1606) -> (24.6951, -77.1606)
  line L11072 (27.3751, -77.1606) -> (27.3751, -76.5606)
  line L11073 (27.5951, -77.1606) -> (27.3751, -77.1606)
  line L11074 (27.3751, -76.5606) -> (27.5951, -76.5606)
  line L11075 (27.5951, -76.5606) -> (27.5951, -77.1606)
  line L11076 (43.7451, -77.1606) -> (43.7451, -76.5606)
  line L11077 (43.5251, -77.1606) -> (43.7451, -77.1606)
  line L11078 (43.7451, -76.5606) -> (43.5251, -76.5606)
  line L11079 (43.5251, -76.5606) -> (43.5251, -77.1606)
  line L11080 (46.4251, -77.1606) -> (46.4251, -76.5606)
  line L11081 (46.6451, -77.1606) -> (46.4251, -77.1606)
  line L11082 (46.6451, -76.5606) -> (46.6451, -77.1606)
  line L11083 (46.4251, -76.5606) -> (46.6451, -76.5606)
  line L11084 (62.5751, -19.385) -> (62.5751, -19.985)
  line L11085 (62.5751, -19.985) -> (62.7951, -19.985)
  line L11086 (62.7951, -19.385) -> (62.5751, -19.385)
  line L11087 (62.7951, -19.985) -> (62.7951, -19.385)
  line L11088 (65.6951, -19.985) -> (65.4751, -19.985)
  line L11089 (65.4751, -19.385) -> (65.6951, -19.385)
  line L11090 (65.4751, -19.985) -> (65.4751, -19.385)
  line L11091 (65.6951, -19.385) -> (65.6951, -19.985)
  line L11092 (62.7951, -76.5606) -> (62.5751, -76.5606)
  line L11093 (62.5751, -76.5606) -> (62.5751, -77.1606)
  line L11094 (62.7951, -77.1606) -> (62.7951, -76.5606)
  line L11095 (62.5751, -77.1606) -> (62.7951, -77.1606)
  line L11096 (65.4751, -76.5606) -> (65.6951, -76.5606)
  line L11097 (65.4751, -77.1606) -> (65.4751, -76.5606)
  line L11098 (65.6951, -77.1606) -> (65.4751, -77.1606)
  line L11099 (65.6951, -76.5606) -> (65.6951, -77.1606)
  line L11100 (62.7951, -38.4351) -> (62.5751, -38.4351)
  line L11101 (62.5751, -39.0351) -> (62.7951, -39.0351)
  line L11102 (62.7951, -39.0351) -> (62.7951, -38.4351)
  line L11103 (62.5751, -38.4351) -> (62.5751, -39.0351)
  line L11104 (65.6951, -39.0351) -> (65.4751, -39.0351)
  line L11105 (65.4751, -39.0351) -> (65.4751, -38.4351)
  line L11106 (65.6951, -38.4351) -> (65.6951, -39.0351)
  line L11107 (65.4751, -38.4351) -> (65.6951, -38.4351)
  line L11108 (62.5751, -57.4978) -> (62.5751, -58.0978)
  line L11109 (62.7951, -58.0978) -> (62.7951, -57.4978)
  line L11110 (62.7951, -57.4978) -> (62.5751, -57.4978)
  line L11111 (62.5751, -58.0978) -> (62.7951, -58.0978)
  line L11112 (65.4751, -58.0978) -> (65.4751, -57.4978)
  line L11113 (65.4751, -57.4978) -> (65.6951, -57.4978)
  line L11114 (65.6951, -58.0978) -> (65.4751, -58.0978)
  line L11115 (65.6951, -57.4978) -> (65.6951, -58.0978)
  line L11116 (81.6252, -38.4351) -> (81.6252, -39.0351)
  line L11117 (81.8452, -39.0351) -> (81.8452, -38.4351)
  line L11118 (81.8452, -38.4351) -> (81.6252, -38.4351)
  line L11119 (81.6252, -39.0351) -> (81.8452, -39.0351)
  line L11120 (84.7452, -38.4351) -> (84.7452, -39.0351)
  line L11121 (84.5252, -39.0351) -> (84.5252, -38.4351)
  line L11122 (84.7452, -39.0351) -> (84.5252, -39.0351)
  line L11123 (84.5252, -38.4351) -> (84.7452, -38.4351)
  line L11124 (81.6252, -77.1606) -> (81.8452, -77.1606)
  line L11125 (81.8452, -76.5606) -> (81.6252, -76.5606)
  line L11126 (81.8452, -77.1606) -> (81.8452, -76.5606)
  line L11127 (81.6252, -76.5606) -> (81.6252, -77.1606)
  line L11128 (84.5252, -77.1606) -> (84.5252, -76.5606)
  line L11129 (84.7452, -76.5606) -> (84.7452, -77.1606)
  line L11130 (84.7452, -77.1606) -> (84.5252, -77.1606)
  line L11131 (84.5252, -76.5606) -> (84.7452, -76.5606)
  line L11132 (81.6252, -19.385) -> (81.6252, -19.985)
  line L11133 (81.8452, -19.385) -> (81.6252, -19.385)
  line L11134 (81.6252, -19.985) -> (81.8452, -19.985)
  line L11135 (81.8452, -19.985) -> (81.8452, -19.385)
  line L11136 (84.5252, -19.985) -> (84.5252, -19.385)
  line L11137 (84.5252, -19.385) -> (84.7452, -19.385)
  line L11138 (84.7452, -19.385) -> (84.7452, -19.985)
  line L11139 (84.7452, -19.985) -> (84.5252, -19.985)
  line L11140 (81.8452, -58.0978) -> (81.8452, -57.4978)
  line L11141 (81.6252, -58.0978) -> (81.8452, -58.0978)
  line L11142 (81.8452, -57.4978) -> (81.6252, -57.4978)
  line L11143 (81.6252, -57.4978) -> (81.6252, -58.0978)
  line L11144 (84.5252, -57.4978) -> (84.7452, -57.4978)
  line L11145 (84.7452, -57.4978) -> (84.7452, -58.0978)
  line L11146 (84.5252, -58.0978) -> (84.5252, -57.4978)
  line L11147 (84.7452, -58.0978) -> (84.5252, -58.0978)
  line L11148 (5.425, -57.4978) -> (5.425, -58.0978)
  line L11149 (5.425, -58.0978) -> (5.645, -58.0978)
  line L11150 (5.645, -57.4978) -> (5.425, -57.4978)
  line L11151 (5.645, -58.0978) -> (5.645, -57.4978)
  line L11152 (8.545, -58.0978) -> (8.325, -58.0978)
  line L11153 (8.325, -57.4978) -> (8.545, -57.4978)
  line L11154 (8.325, -58.0978) -> (8.325, -57.4978)
  line L11155 (8.545, -57.4978) -> (8.545, -58.0978)
  line L11156 (5.645, -19.985) -> (5.645, -19.385)
  line L11157 (5.425, -19.385) -> (5.425, -19.985)
  line L11158 (5.645, -19.385) -> (5.425, -19.385)
  line L11159 (5.425, -19.985) -> (5.645, -19.985)
  line L11160 (8.545, -19.985) -> (8.325, -19.985)
  line L11161 (8.325, -19.385) -> (8.545, -19.385)
  line L11162 (8.545, -19.385) -> (8.545, -19.985)
  line L11163 (8.325, -19.985) -> (8.325, -19.385)
  line L11164 (5.425, -38.4351) -> (5.425, -39.0351)
  line L11165 (5.425, -39.0351) -> (5.645, -39.0351)
  line L11166 (5.645, -38.4351) -> (5.425, -38.4351)
  line L11167 (5.645, -39.0351) -> (5.645, -38.4351)
  line L11168 (8.545, -39.0351) -> (8.325, -39.0351)
  line L11169 (8.325, -39.0351) -> (8.325, -38.4351)
  line L11170 (8.545, -38.4351) -> (8.545, -39.0351)
  line L11171 (8.325, -38.4351) -> (8.545, -38.4351)
  line L11172 (24.6951, -39.0351) -> (24.6951, -38.4351)
  line L11173 (24.4751, -39.0351) -> (24.6951, -39.0351)
  line L11174 (24.6951, -38.4351) -> (24.4751, -38.4351)
  line L11175 (24.4751, -38.4351) -> (24.4751, -39.0351)
  line L11176 (27.3751, -38.4351) -> (27.5951, -38.4351)
  line L11177 (27.3751, -39.0351) -> (27.3751, -38.4351)
  line L11178 (27.5951, -38.4351) -> (27.5951, -39.0351)
  line L11179 (27.5951, -39.0351) -> (27.3751, -39.0351)
  line L11180 (24.4751, -19.985) -> (24.6951, -19.985)
  line L11181 (24.6951, -19.385) -> (24.4751, -19.385)
  line L11182 (24.6951, -19.985) -> (24.6951, -19.385)
  line L11183 (24.4751, -19.385) -> (24.4751, -19.985)
  line L11184 (27.3751, -19.385) -> (27.5951, -19.385)
  line L11185 (27.5951, -19.385) -> (27.5951, -19.985)
  line L11186 (27.5951, -19.985) -> (27.3751, -19.985)
  line L11187 (27.3751, -19.985) -> (27.3751, -19.385)
  line L11188 (24.6951, -57.4978) -> (24.4751, -57.4978)
  line L11189 (24.4751, -58.0978) -> (24.6951, -58.0978)
  line L11190 (24.6951, -58.0978) -> (24.6951, -57.4978)
  line L11191 (24.4751, -57.4978) -> (24.4751, -58.0978)
  line L11192 (27.5951, -58.0978) -> (27.3751, -58.0978)
  line L11193 (27.3751, -57.4978) -> (27.5951, -57.4978)
  line L11194 (27.3751, -58.0978) -> (27.3751, -57.4978)
  line L11195 (27.5951, -57.4978) -> (27.5951, -58.0978)
  line L11196 (43.7451, -19.985) -> (43.7451, -19.385)
  line L11197 (43.5251, -19.985) -> (43.7451, -19.985)
  line L11198 (43.7451, -19.385) -> (43.5251, -19.385)
  line L11199 (43.5251, -19.385) -> (43.5251, -19.985)
  line L11200 (46.4251, -19.985) -> (46.4251, -19.385)
  line L11201 (46.6451, -19.385) -> (46.6451, -19.985)
  line L11202 (46.4251, -19.385) -> (46.6451, -19.385)
  line L11203 (46.6451, -19.985) -> (46.4251, -19.985)
  line L11204 (43.7451, -57.4978) -> (43.5251, -57.4978)
  line L11205 (43.7451, -58.0978) -> (43.7451, -57.4978)
  line L11206 (43.5251, -58.0978) -> (43.7451, -58.0978)
  line L11207 (43.5251, -57.4978) -> (43.5251, -58.0978)
  line L11208 (46.4251, -57.4978) -> (46.6451, -57.4978)
  line L11209 (46.6451, -58.0978) -> (46.4251, -58.0978)
  line L11210 (46.6451, -57.4978) -> (46.6451, -58.0978)
  line L11211 (46.4251, -58.0978) -> (46.4251, -57.4978)
  line L11212 (43.5251, -39.0351) -> (43.7451, -39.0351)
  line L11213 (43.7451, -38.4351) -> (43.5251, -38.4351)
  line L11214 (43.5251, -38.4351) -> (43.5251, -39.0351)
  line L11215 (43.7451, -39.0351) -> (43.7451, -38.4351)
  line L11216 (46.4251, -38.4351) -> (46.6451, -38.4351)
  line L11217 (46.6451, -38.4351) -> (46.6451, -39.0351)
  line L11218 (46.4251, -39.0351) -> (46.4251, -38.4351)
  line L11219 (46.6451, -39.0351) -> (46.4251, -39.0351)
  line L11220 (214.9754, -19.385) -> (214.9754, -19.985)
  line L11221 (214.9754, -19.985) -> (215.1954, -19.985)
  line L11222 (215.1954, -19.985) -> (215.1954, -19.385)
  line L11223 (215.1954, -19.385) -> (214.9754, -19.385)
  line L11224 (217.8754, -19.985) -> (217.8754, -19.385)
  line L11225 (217.8754, -19.385) -> (218.0954, -19.385)
  line L11226 (218.0954, -19.985) -> (217.8754, -19.985)
  line L11227 (218.0954, -19.385) -> (218.0954, -19.985)
  line L11228 (214.9754, -76.5606) -> (214.9754, -77.1606)
  line L11229 (215.1954, -77.1606) -> (215.1954, -76.5606)
  line L11230 (214.9754, -77.1606) -> (215.1954, -77.1606)
  line L11231 (215.1954, -76.5606) -> (214.9754, -76.5606)
  line L11232 (217.8754, -76.5606) -> (218.0954, -76.5606)
  line L11233 (218.0954, -77.1606) -> (217.8754, -77.1606)
  line L11234 (218.0954, -76.5606) -> (218.0954, -77.1606)
  line L11235 (217.8754, -77.1606) -> (217.8754, -76.5606)
  line L11236 (214.9754, -58.0978) -> (215.1954, -58.0978)
  line L11237 (215.1954, -58.0978) -> (215.1954, -57.4978)
  line L11238 (215.1954, -57.4978) -> (214.9754, -57.4978)
  line L11239 (214.9754, -57.4978) -> (214.9754, -58.0978)
  line L11240 (217.8754, -57.4978) -> (218.0954, -57.4978)
  line L11241 (218.0954, -57.4978) -> (218.0954, -58.0978)
  line L11242 (218.0954, -58.0978) -> (217.8754, -58.0978)
  line L11243 (217.8754, -58.0978) -> (217.8754, -57.4978)
  line L11244 (214.9754, -39.0351) -> (215.1954, -39.0351)
  line L11245 (214.9754, -38.4351) -> (214.9754, -39.0351)
  line L11246 (215.1954, -38.4351) -> (214.9754, -38.4351)
  line L11247 (215.1954, -39.0351) -> (215.1954, -38.4351)
  line L11248 (217.8754, -39.0351) -> (217.8754, -38.4351)
  line L11249 (218.0954, -38.4351) -> (218.0954, -39.0351)
  line L11250 (217.8754, -38.4351) -> (218.0954, -38.4351)
  line L11251 (218.0954, -39.0351) -> (217.8754, -39.0351)
  line L11252 (195.9254, -38.4351) -> (195.9254, -39.0351)
  line L11253 (195.9254, -39.0351) -> (196.1454, -39.0351)
  line L11254 (196.1454, -39.0351) -> (196.1454, -38.4351)
  line L11255 (196.1454, -38.4351) -> (195.9254, -38.4351)
  line L11256 (198.8254, -38.4351) -> (199.0454, -38.4351)
  line L11257 (199.0454, -38.4351) -> (199.0454, -39.0351)
  line L11258 (199.0454, -39.0351) -> (198.8254, -39.0351)
  line L11259 (198.8254, -39.0351) -> (198.8254, -38.4351)
  line L11260 (196.1454, -76.5606) -> (195.9254, -76.5606)
  line L11261 (195.9254, -76.5606) -> (195.9254, -77.1606)
  line L11262 (196.1454, -77.1606) -> (196.1454, -76.5606)
  line L11263 (195.9254, -77.1606) -> (196.1454, -77.1606)
  line L11264 (199.0454, -77.1606) -> (198.8254, -77.1606)
  line L11265 (199.0454, -76.5606) -> (199.0454, -77.1606)
  line L11266 (198.8254, -77.1606) -> (198.8254, -76.5606)
  line L11267 (198.8254, -76.5606) -> (199.0454, -76.5606)
  line L11268 (195.9254, -57.4978) -> (195.9254, -58.0978)
  line L11269 (196.1454, -58.0978) -> (196.1454, -57.4978)
  line L11270 (195.9254, -58.0978) -> (196.1454, -58.0978)
  line L11271 (196.1454, -57.4978) -> (195.9254, -57.4978)
  line L11272 (198.8254, -57.4978) -> (199.0454, -57.4978)
  line L11273 (199.0454, -58.0978) -> (198.8254, -58.0978)
  line L11274 (199.0454, -57.4978) -> (199.0454, -58.0978)
  line L11275 (198.8254, -58.0978) -> (198.8254, -57.4978)
  line L11276 (195.9254, -19.385) -> (195.9254, -19.985)
  line L11277 (196.1454, -19.385) -> (195.9254, -19.385)
  line L11278 (195.9254, -19.985) -> (196.1454, -19.985)
  line L11279 (196.1454, -19.985) -> (196.1454, -19.385)
  line L11280 (198.8254, -19.985) -> (198.8254, -19.385)
  line L11281 (199.0454, -19.385) -> (199.0454, -19.985)
  line L11282 (199.0454, -19.985) -> (198.8254, -19.985)
  line L11283 (198.8254, -19.385) -> (199.0454, -19.385)
  line L11284 (196.9422, -3.67) -> (197.1272, -3.67)
  line L11285 (197.1272, -3.67) -> (197.1272, -3.92)
  line L11286 (197.1272, -3.92) -> (196.9422, -3.92)
  line L11287 (196.9422, -3.92) -> (196.9422, -3.67)
  line L11288 (196.9421, -4.97) -> (197.1271, -4.97)
  line L11289 (196.9421, -5.22) -> (196.9421, -4.97)
  line L11290 (197.1271, -5.22) -> (196.9421, -5.22)
  line L11291 (197.1271, -4.97) -> (197.1271, -5.22)
  line L11292 (195.5424, -3.92) -> (195.5424, -3.67)
  line L11293 (195.7274, -3.67) -> (195.7274, -3.92)
  line L11294 (195.7274, -3.92) -> (195.5424, -3.92)
  line L11295 (195.5424, -3.67) -> (195.7274, -3.67)
  line L11296 (195.7274, -4.32) -> (195.7274, -4.57)
  line L11297 (195.7274, -4.57) -> (195.5424, -4.57)
  line L11298 (195.5424, -4.57) -> (195.5424, -4.32)
  line L11299 (195.5424, -4.32) -> (195.7274, -4.32)
  line L11300 (195.5424, -4.97) -> (195.7274, -4.97)
  line L11301 (195.7274, -4.97) -> (195.7274, -5.22)
  line L11302 (195.7274, -5.22) -> (195.5424, -5.22)
  line L11303 (195.5424, -5.22) -> (195.5424, -4.97)
  line L11304 (208.6954, -3.4061) -> (208.2754, -3.4061)
  line L11305 (208.2754, -3.4061) -> (208.2754, -3.1661)
  line L11306 (208.2754, -3.1661) -> (208.6954, -3.1661)
  line L11307 (208.6954, -3.1661) -> (208.6954, -3.4061)
  line L11308 (208.6954, -2.906) -> (208.2754, -2.906)
  line L11309 (208.2754, -2.906) -> (208.2754, -2.666)
  line L11310 (208.6954, -2.666) -> (208.6954, -2.906)
  line L11311 (208.2754, -2.666) -> (208.6954, -2.666)
  line L11312 (208.2754, -2.4059) -> (208.2754, -2.1659)
  line L11313 (208.2754, -2.1659) -> (208.6954, -2.1659)
  line L11314 (208.6954, -2.1659) -> (208.6954, -2.4059)
  line L11315 (208.6954, -2.4059) -> (208.2754, -2.4059)
  line L11316 (208.2754, -1.906) -> (208.2754, -1.666)
  line L11317 (208.6954, -1.666) -> (208.6954, -1.906)
  line L11318 (208.6954, -1.906) -> (208.2754, -1.906)
  line L11319 (208.2754, -1.666) -> (208.6954, -1.666)
  line L11320 (208.2754, -1.4061) -> (208.2754, -1.1661)
  line L11321 (208.2754, -1.1661) -> (208.6954, -1.1661)
  line L11322 (208.6954, -1.1661) -> (208.6954, -1.4061)
  line L11323 (208.6954, -1.4061) -> (208.2754, -1.4061)
  line L11324 (211.6754, -1.1659) -> (212.0954, -1.1659)
  line L11325 (211.6754, -1.4059) -> (211.6754, -1.1659)
  line L11326 (212.0954, -1.4059) -> (211.6754, -1.4059)
  line L11327 (212.0954, -1.1659) -> (212.0954, -1.4059)
  line L11328 (212.0954, -1.906) -> (211.6754, -1.906)
  line L11329 (211.6754, -1.906) -> (211.6754, -1.666)